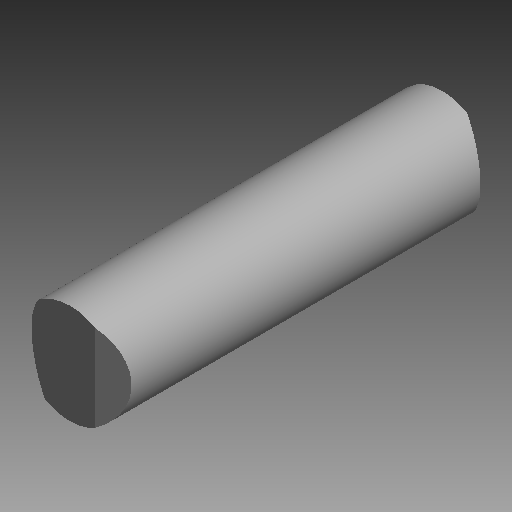
# Autodesk Inventor part: 06B - 1 RP- Pin 1
Saved by Autodesk Inventor 2019 (Build 230136000, 136)
## iProperties
Category: PARTsolutions
Company: KANA
Part Number: 06B - 1 RP- Pin 1
Material: 一般
Catalog Web Link: www.cadenas.de
Description: Standard Chain Pin-
Vendor: KANA
Document SubType Name: Modeling
Designer: partserver
Manufacturer: KANA
Mass: 0.102049 g
Surface Area: 1.39861 cm^2
Volume: 0.102049 cm^3
Density: 1 g/cm^3
Appearance: PSOLRGB-192-192-192
PSOL_IDENT_0: {$CADENAS_DATA\23d-libs\kana\roller_chain\standard_chain\standard_chain_body2.prj},185 {VTYP=3D},{NB=
PSOL_IDENT_1: 06B - 1 RP- Pin 1},{LINA=06B - 1 RP},{NN=Standard Chain Pin},{DATE=04.07.2018 01:10:23},{GEOMDATE=13
PSOL_IDENT_2: .09.2016 07:09:00},{VERSION=},{LINEID=60},{WBVAR=NOL},{WBNUMERIC=NOL}  {NB=06B - 1 RP- Pin 1},{LINA=
PSOL_IDENT_3: 06B - 1 RP},{KT=DUMMY},{CNO=06B},{PT=RP},{NOL=1},{NOLX=1},{P=9.525},{R=6.350},{W=5.720},{T=1.000},{H=
PSOL_IDENT_4: 8.100},{D=3.280},{L=13.6},{C=10.24},{VERS1=1.000},{L1=6.1},{L2=7.5},{L3=12.2},{C11=0},{VERS2=1}
NB: 06B - 1 RP- Pin 1
NN: Standard Chain Pin
NBSYN: $CNO. - $NOL. $PT.- Pin 1
LINA: 06B - 1 RP
CATALOG: KANA
CNO: 06B
PT: RP
NOL: 1
P: 9.525
R: 6.35
W: 5.72
T: 1
H: 8.1
D: 3.28
VERS1: 1
VERS2: 1
SUPPLIER: KANA
ARTICLENO: 06B - 1 RP- Pin 1
BOMINFO: 06B - 1 RP
CREATOR: CADENAS GmbH
Title: 06B - 1 RP
Author: Cadenas PARTsolutions
Autodesk Inventor part; units mm, degrees
sketch "Sketch_1" plane through (0, 0, 0) normal (0, 0, 1) x (1, 0, 0)
  line L0 (0, -6.1) -> (0, 6.1)
  line L1 (0, 6.1) -> (1.64, 6.1)
  line L2 (1.64, 6.1) -> (1.64, -6.1)
  line L3 (1.64, -6.1) -> (0, -6.1)
  line L4 (0, -6.1) -> (0, 6.1)
  constraints: 10 end point
revolve "Revolution1" add sketch "Sketch_1" angle 360 about axis through (0, -6.1, 0) along (0, -1, 0)
sketch "Sketch_7" plane through (0, 0, 0) normal (0, 0, 1) x (1, 0, 0)
  line L0 (0.82, 6.1) -> (2.46, 5.3353)
  line L1 (2.46, 5.3353) -> (2.46, 6.92)
  line L2 (2.46, 6.92) -> (0.82, 6.92)
  line L3 (0.82, 6.92) -> (0.82, 6.1)
  constraints: 8 end point
extrude "Extrusion1" cut sketch "Sketch_7" along normal mid plane 3.28
sketch "Sketch_8" plane through (0, 0, 0) normal (0, 0, 1) x (1, 0, 0)
  line L0 (-2.46, 6.92) -> (-2.46, 5.3353)
  line L1 (-2.46, 5.3353) -> (-0.82, 6.1)
  line L2 (-0.82, 6.1) -> (-0.82, 6.92)
  line L3 (-0.82, 6.92) -> (-2.46, 6.92)
  constraints: 8 end point
extrude "Extrusion2" cut sketch "Sketch_8" along normal mid plane 3.28
sketch "Sketch_9" plane through (0, 0, 0) normal (0, 0, 1) x (1, 0, 0)
  line L0 (0.82, -6.1) -> (0.82, -6.92)
  line L1 (0.82, -6.92) -> (2.46, -6.92)
  line L2 (2.46, -6.92) -> (2.46, -5.3353)
  line L3 (2.46, -5.3353) -> (0.82, -6.1)
  constraints: 8 end point
extrude "Extrusion3" cut sketch "Sketch_9" along normal mid plane 3.28
sketch "Sketch_10" plane through (0, 0, 0) normal (0, 0, 1) x (1, 0, 0)
  line L0 (-2.46, -6.92) -> (-0.82, -6.92)
  line L1 (-0.82, -6.92) -> (-0.82, -6.1)
  line L2 (-0.82, -6.1) -> (-2.46, -5.3353)
  line L3 (-2.46, -5.3353) -> (-2.46, -6.92)
  constraints: 8 end point
extrude "Extrusion4" cut sketch "Sketch_10" along normal mid plane 3.28
ref_plane "Body2_1_XY" through (0, 0, 0) normal (0, 1, 0) x (1, 0, 0)
ref_plane "Body2_1_YZ" through (0, 0, 0) normal (1, 0, 0) x (0, 0, -1)
ref_plane "Body2_1_ZX" through (0, 0, 0) normal (0, 0, -1) x (0, 1, 0)
ref_plane "for_pin_XY" through (0, -5.3803, 0) normal (1, 0, 0) x (0, 0, -1)
ref_plane "for_pin_YZ" through (0, -5.3803, 0) normal (0, 0, -1) x (0, 1, 0)
ref_plane "for_pin_ZX" through (0, -5.3803, 0) normal (0, 1, 0) x (1, 0, 0)
ref_plane "to_dummy_1_XY" through (0, 0, 0) normal (0, -1, 0) x (1, 0, 0)
ref_plane "to_dummy_1_YZ" through (0, 0, 0) normal (1, 0, 0) x (0, 0, 1)
ref_plane "to_dummy_1_ZX" through (0, 0, 0) normal (0, 0, 1) x (0, -1, 0)
body "Solid1"
